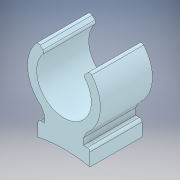
# Autodesk Inventor part: snap_grip
Saved by Autodesk Inventor 2018 (Build 220112000, 112)
## iProperties
Created: 2018-09-02
Part Number: snap_grip
Material: Generic
Document SubType Name: Modeling
Designer: Fredy Espana C
Density: 1 g/cm^3
Appearance: Default
Author: Fredy Espana C
Autodesk Inventor part; units mm, degrees
ref_plane "YZ Plane" through (0, 0, 0) normal (1, 0, 0) x (0, 1, 0)
ref_plane "XZ Plane" through (0, 0, 0) normal (0, 1, 0) x (-1, 0, 0)
ref_plane "XY Plane" through (0, 0, 0) normal (0, 0, 1) x (1, 0, 0)
sketch "Sketch1" plane through (0, 0, 0) normal (1, 0, 0) x (0, 1, 0)
  arc A0 (3.7123, 3.7123) -> (3.7123, -3.7123) centre (0, 0) ccw
  line L0 (-5.9108, 3.75) -> (-7.9108, 3.75)
  line L1 (-7.9108, -3.75) -> (-5.9108, -3.75)
  line L2 (3.7123, -3.7123) -> (4.9497, -4.9497)
  line L3 (3.7123, 3.7123) -> (4.9497, 4.9497)
  arc A1 (-5.9108, -3.75) -> (4.9497, -4.9497) centre (0, 0) ccw
  arc A2 (4.9497, 4.9497) -> (-5.9108, 3.75) centre (0, 0) ccw
  line L4 (4.9497, 4.9497) -> (0, 0) construction
  line L5 (0, 0) -> (4.9497, -4.9497) construction
  line L6 (-7.9108, 5) -> (-10.9108, 5)
  line L7 (-10.9108, -5) -> (-7.9108, -5)
  line L8 (-7.9108, -5) -> (-7.9108, -3.75)
  line L9 (-7.9108, 3.75) -> (-7.9108, 5)
  arc A3 (-10.9108, -5) -> (-10.9108, 5) centre (-35.8138, 0) ccw
  line L10 (-7.9108, 3.75) -> (-7.9108, -3.75) construction
  point P0 (-5.25, 0)
  point P1 (-13.9108, 0)
  point P2 (-7.9108, 4.375)
  point P3 (-7.9108, -4.375)
  point P4 (-7.9108, 0)
  dimension "d0" = 90
  dimension "d5" = 2
  dimension "d9" = 14
  dimension "d10" = 10.5
  dimension "d11" = 7.5
  dimension "d12" = 3
  dimension "d14" = 50.8
  dimension "d15" = 10
  constraints: 22 end point, 9 point on circle, 4 centre point, 3 coincident, 3 equal length, 3 midpoint, 2 horizontal, 2 horizontal alignment, 2 parallel, 2 perpendicular, 2 vertical alignment, 1 concentric, 1 vertical
  measures "d0" angle of L3 L2
  measures "d5" distance of L1.start L1.end
  measures "d9" diameter of A1
  measures "d10" diameter of A0
  measures "d11" distance between parallel lines of L1 L0
  measures "d12" distance of L7.start L7.end
  measures "d14" diameter of A3
  measures "d15" distance between parallel lines of L7 L6
extrude "Extrusion1" add sketch "Sketch1" along normal blind 10
fillet "Fillet1" radius 0.5 6 edges at (5, -7.9108, -5) (5, 4.9497, -4.9497) (5, 4.9497, 4.9497) (5, 3.7123, 3.7123) (5, 3.7123, -3.7123) (5, -7.9108, 5)
chamfer "Chamfer1" distance 0.75 angle 45 2 edges at (5, -5.9108, 3.75) (5, -5.9108, -3.75)
body "Solid1"
